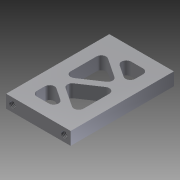
# Autodesk Inventor part: upper gearbox stand off standard
Saved by Autodesk Inventor 2012 (Build 160160000, 160)
## iProperties
Created: 2012-08-28
Part Number: upper gearbox stand off standard
Material: Default
Document SubType Name: Modeling
Designer: Team-2471
Density: 1 g/cm^3
Author: Team-2471
Autodesk Inventor part; units mm, degrees
ref_plane "YZ Plane" through (0, 0, 0) normal (1, 0, 0) x (0, 1, 0)
ref_plane "XZ Plane" through (0, 0, 0) normal (0, 1, 0) x (-1, 0, 0)
sketch "Sketch1" plane through (0, 0, 0) normal (0, 0, 1) x (1, 0, 0)
  line L0 (0, 0) -> (31.75, 0)
  line L1 (31.75, 0) -> (31.75, 6.35)
  line L2 (31.75, 6.35) -> (0, 6.35)
  line L3 (0, 6.35) -> (0, 0)
  point P0 (3.175, 3.175)
  point P1 (28.575, 3.175)
  dimension "d0" = 6.35
  dimension "d1" = 31.75
  dimension "d4" = 3.175
  dimension "d5" = 3.175
  dimension "d6" = 3.175
  dimension "d8" = 3.175
  constraints: 8 end point, 2 parallel, 1 horizontal, 1 perpendicular
  measures "d0" distance between parallel lines of L0 L2
  measures "d1" distance of L1.end L2.end
  measures "d4" distance from line of L3 point (3.175, 3.175)
  measures "d5" distance from line of L0 point (3.175, 3.175)
  measures "d6" distance from line of L2 point (28.575, 3.175)
  measures "d8" distance from line of L1 point (28.575, 3.175)
extrude "Extrusion1" add sketch "Sketch1" along normal blind 50.8
sketch "Sketch2" plane through (0, 0, 50.8) normal (0, 0, 1) x (1, 0, 0)
  circle A0 centre (3.175, 3.175) radius 1.5875 projected
  circle A1 centre (28.575, 3.175) radius 1.5875 projected
ref_plane "Work Plane1" through (0, 3.175, 0) normal (0, 1, 0) x (1, 0, 0)
sketch "Sketch3" plane through (0, 3.175, 0) normal (0, 1, 0) x (1, 0, 0)
  line L0 (0, 0) -> (31.75, 0) projected
  line L1 (0, 0) -> (0, -50.8) projected
  line L2 (31.75, 0) -> (31.75, -50.8) projected
  line L3 (31.75, -50.8) -> (0, -50.8) projected
  line L4 (6.35, -6.35) -> (25.4, -6.35)
  line L5 (25.4, -6.35) -> (25.4, -44.45)
  line L6 (25.4, -44.45) -> (6.35, -44.45)
  line L7 (6.35, -44.45) -> (6.35, -6.35)
  line L8 (25.4, -44.45) -> (6.35, -31.75) construction
  line L9 (25.4, -19.05) -> (6.35, -6.35) construction
  line L10 (6.35, -31.75) -> (25.4, -19.05) construction
  line L11 (22.5381, -44.45) -> (6.35, -33.6579)
  line L12 (25.4, -42.5421) -> (9.2119, -31.75)
  line L13 (9.2119, -31.75) -> (25.4, -20.9579)
  line L14 (6.35, -29.8421) -> (22.5381, -19.05)
  line L15 (22.5381, -19.05) -> (6.35, -8.2579)
  line L16 (25.4, -17.1421) -> (9.2119, -6.35)
  point P0 (25.4, -15.6798)
  point P1 (6.35, -19.8802)
  point P2 (6.35, -8.0598)
  point P3 (10.6245, -6.35)
  point P4 (25.4, -12.2602)
  dimension "d27" = 6.35
  dimension "d28" = 6.35
  dimension "d29" = 6.35
  dimension "d30" = 6.35
  dimension "d31" = 33.69
  dimension "d32" = 67.38
  dimension "d33" = 1.5875
  dimension "d34" = 3.175
  dimension "d35" = 1.5875
  dimension "d36" = 3.175
  dimension "d37" = 1.5875
  dimension "d38" = 3.175
  constraints: 26 end point, 15 point on line, 7 parallel, 1 horizontal, 1 perpendicular
  measures "d27" distance between parallel lines of L3 L6
  measures "d28" distance between parallel lines of L0 L4
  measures "d29" distance between parallel lines of L1 L7
  measures "d30" distance between parallel lines of L2 L5
  measures "d31" angle of L6 L8
  measures "d32" angle of L8 L10
  measures "d33" distance between parallel lines of L8 L11
  measures "d34" distance between parallel lines of L11 L12
  measures "d35" distance between parallel lines of L10 L13
  measures "d36" distance between parallel lines of L14 L13
  measures "d37" distance between parallel lines of L9 L15
  measures "d38" distance between parallel lines of L15 L16
extrude "Extrusion4" cut sketch "Sketch3" along normal mid plane 25.4 contours L4 L5 L16 | L15 L14 L7 | L5 L12 L13 | L11 L6 L7
sketch "Sketch5" plane through (0, 6.35, 0) normal (0, 1, 0) x (1, 0, 0)
  line L0 (0, -50.8) -> (31.75, -50.8) projected
  line L1 (31.75, 0) -> (31.75, -50.8) projected
  line L2 (0, 0) -> (31.75, 0)
  line L3 (31.75, 0) -> (31.75, -6.35)
  line L4 (31.75, -6.35) -> (0, -6.35)
  line L5 (0, -6.35) -> (0, 0)
  line L6 (0, -6.35) -> (31.75, -6.35)
  line L7 (31.75, -6.35) -> (31.75, -44.45)
  line L8 (31.75, -44.45) -> (0, -44.45)
  line L9 (0, -44.45) -> (0, -6.35)
  line L10 (31.75, -44.45) -> (0, -44.45)
  line L11 (0, -44.45) -> (0, -50.8)
  line L12 (0, -50.8) -> (31.75, -50.8)
  line L13 (31.75, -50.8) -> (31.75, -44.45)
  constraints: 24 end point, 6 parallel, 3 horizontal, 3 perpendicular, 2 point on line
extrude "Extrusion6" cut sketch "Sketch5" against normal blind 1.5875 contours L9 L4 L1 L8
sketch "Sketch6" plane through (0, 0, 0) normal (0, -1, 0) x (1, 0, 0)
  line L0 (0, 0) -> (0, 50.8) projected
  line L1 (31.75, 0) -> (31.75, 50.8) projected
  line L2 (0, 50.8) -> (31.75, 50.8)
  line L3 (31.75, 50.8) -> (31.75, 44.45)
  line L4 (31.75, 44.45) -> (0, 44.45)
  line L5 (0, 44.45) -> (0, 50.8)
  line L6 (31.75, 44.45) -> (0, 44.45)
  line L7 (0, 44.45) -> (0, 6.35)
  line L8 (0, 6.35) -> (31.75, 6.35)
  line L9 (31.75, 6.35) -> (31.75, 44.45)
  line L10 (31.75, 0) -> (0, 0)
  line L11 (0, 0) -> (0, 6.35)
  line L12 (0, 6.35) -> (31.75, 6.35)
  line L13 (31.75, 6.35) -> (31.75, 0)
  constraints: 24 end point, 6 parallel, 3 horizontal, 3 perpendicular, 2 point on line
extrude "Extrusion8" cut sketch "Sketch6" against normal blind 1.5875 contours L0 L4 L1 L8
extrude "Extrusion11" add sketch "Sketch3" along normal mid plane 6.35 contours L0 L2 L3 L1 | L4 L16 L5 L13 L12 L6 L11 L7 L14 L15
fillet "Fillet7" radius 2.3813 12 edges at (25.4, 3.175, 17.1421) (22.5381, 3.175, 19.05) (25.4, 3.175, 20.9579) (25.4, 3.175, 42.5421) (22.5381, 3.175, 44.45) (6.35, 3.175, 44.45) (6.35, 3.175, 33.6579) (9.2119, 3.175, 31.75) (6.35, 3.175, 29.8421) (6.35, 3.175, 8.2579) (9.2119, 3.175, 6.35) (25.4, 3.175, 6.35)
extrude "Extrusion12" cut sketch "Sketch2" against normal blind 12.7
hole "Hole2" at (3.175, 3.175, 0) at (28.575, 3.175, 0) direction (0, 0, 1) diameter 3.175 depth 12.7 tip angle 118
thread "Thread5" size "5-40 UNC" class "2B" standard "ANSI Unified Screw Threads" full length
thread "Thread6" size "5-40 UNC" class "2B" standard "ANSI Unified Screw Threads" full length
thread "Thread7" size "5-40 UNC" class "2B" standard "ANSI Unified Screw Threads" full length
thread "Thread8" size "5-40 UNC" class "2B" standard "ANSI Unified Screw Threads" full length
equation "\"d5\" = d4"
equation "\"d8\" = d4"
equation "\"d28\" = d30"
equation "\"d29\" = d27"
equation "\"d30\" = d29"
equation "\"d32\" = 2 * d31"
equation "\"d34\" = 2 * d33"
equation "\"d35\" = d33"
equation "\"d36\" = d34"
equation "\"d37\" = d35"
equation "\"d38\" = d36"
body "Solid1"
